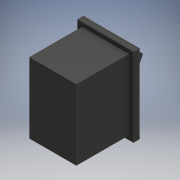
# Autodesk Inventor part: interruptor
Saved by Autodesk Inventor 2017 (Build 210142000, 142)
## iProperties
Part Number: interruptor
Material: Genérico
Document SubType Name: Modeling
Designer: Roberto
Density: 1 g/cm^3
Appearance: Valor por defecto
Author: Roberto
Autodesk Inventor part; units mm, degrees
ref_plane "YZ Plane" through (0, 0, 0) normal (1, 0, 0) x (0, 1, 0)
ref_plane "XZ Plane" through (0, 0, 0) normal (0, 1, 0) x (-1, 0, 0)
ref_plane "XY Plane" through (0, 0, 0) normal (0, 0, 1) x (1, 0, 0)
sketch "Boceto1" plane through (0, 0, 0) normal (0, 1, 0) x (-1, 0, 0)
  line L0 (0, 0) -> (0, -2.08)
  line L1 (0, -2.08) -> (1.48, -2.08)
  line L2 (1.48, -2.08) -> (1.48, 0)
  line L3 (1.48, 0) -> (0, 0)
  dimension "d0" = 2.08
  dimension "d1" = 1.48
  constraints: 8 end point, 3 perpendicular, 1 vertical
  measures "d0" distance of L0.start L0.end
  measures "d1" distance of L0.end L1.end
extrude "Extrusión1" add sketch "Boceto1" along normal blind 0.2
fillet "Empalme1" radius 0.06 4 edges at (0, 0.2, -1.04) (-0.74, 0.2, -2.08) (-1.48, 0.2, -1.04) (-0.74, 0.2, 0)
sketch "Boceto2" plane through (0, 0.2, 0) normal (0, 1, 0) x (1, 0, 0)
  line L0 (-1.48, 2.08) -> (-1.48, 0) projected
  line L1 (0, 2.08) -> (-1.48, 2.08) projected
  line L2 (-1.48, 0) -> (0, 0) projected
  line L3 (0, 2.08) -> (0, 0)
  arc A0 (-0.3478, 1.7532) -> (-1.1148, 1.7481) centre (-0.7208, 0.1817) ccw
  arc A1 (-1.1148, 1.7481) -> (-1.1048, 0.3223) centre (2.5123, 1.0607) ccw
  line L4 (0, 0) -> (-1.48, 0)
  arc A2 (-1.1048, 0.3223) -> (-0.3378, 0.3172) centre (-0.7108, 1.8887) ccw
  arc A3 (-0.3378, 0.3172) -> (-0.3478, 1.7532) centre (-3.6438, 1.0121) ccw
  constraints: 8 point on circle, 4 centre point, 4 end point
extrude "Extrusión2" add sketch "Boceto2" along normal blind 0.4 contours A3 A2 A1 A0
sketch "Boceto3" plane through (0, 0, 0) normal (1, 0, 0) x (0, 1, 0)
  line L0 (0.2, 0.051) -> (0.2, -2.029)
  arc A0 (0.551, -0.4739) -> (0.2, -0.2735) centre (0.0286, -0.9813) ccw
  arc A1 (0.551, -0.4739) -> (0.2, -1.5473) centre (2.2219, -1.6144) ccw
  line L1 (0.2, -2.02) -> (0.2, -0.06) projected
  line L2 (0.2, -0.2735) -> (0.6, -0.2735) projected
  line L3 (0.2, 0.051) -> (0.9906, 0.051)
  line L4 (0.9906, 0.051) -> (0.9906, -2.1784)
  line L5 (0.9906, -2.1784) -> (0.2, -2.1784)
  line L6 (0.2, -2.1784) -> (0.2, -1.5473)
  arc A2 (0.551, -0.4739) -> (0.2, -1.5473) centre (2.2219, -1.6144) ccw
  arc A3 (0.551, -0.4739) -> (0.2, -0.2735) centre (0.0286, -0.9813) ccw
  line L7 (0.2, -0.2735) -> (0.2, 0.051)
  point P0 (0, 0)
  constraints: 12 end point, 8 point on circle, 4 centre point, 3 point on line, 2 perpendicular, 1 collinear, 1 concentric, 1 horizontal, 1 vertical
extrude "Extrusión3" cut sketch "Boceto3" against normal blind 4 contours L3 L4 L5 L6 L0 A1 A0
fillet "Empalme2" radius 0.43 2 edges at (-0.9202, 0.2488, -0.2871) (-0.5128, 0.2442, -0.2857)
sketch "Boceto4" plane through (0, 0, 0) normal (0, -1, 0) x (1, 0, 0)
  line L0 (0, 0) -> (0, -2.08) projected
  line L1 (-1.48, 0) -> (0, 0) projected
  line L2 (-1.48, -2.08) -> (-1.48, 0) projected
  line L3 (0, -2.08) -> (-1.48, -2.08) projected
  line L4 (0, 0) -> (0, -2.08) projected
  line L5 (-0.12, -1.97) -> (-1.36, -1.97)
  line L6 (-1.36, -0.11) -> (-1.36, -1.97)
  line L7 (-0.12, -1.97) -> (-0.12, -0.11)
  line L8 (-1.36, -0.11) -> (-0.12, -0.11)
  constraints: 8 end point, 2 vertical, 1 perpendicular
extrude "Extrusión4" add sketch "Boceto4" along normal blind 1.39 contours L5 L6 L8 L7
